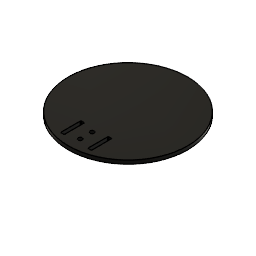
Mirror Mount v1 (Autodesk Fusion 360 design; units mm, degrees)
part number: 2026-03-18-09-30-07-770
Autodesk Fusion 360 part; units mm, degrees
note: some values were not read from the file. Set by a fixed rule: which sketch regions a step uses.
sketch "Sketch1" plane through (0, 0, 0) normal (0, 1, 0) x (1, 0, 0)
  circle A0 centre (0, 0) radius 27.5
  circle A1 centre (0, 0) radius 25
  circle A2 centre (0, 0) radius 50
  circle A3 centre (0, 0) radius 24
  line L0 (0, 0) -> (24, 0)
  dimension "d1" = 55
  dimension "d2" = 50
  dimension "d3" = 100
  dimension "d6" = 48
  constraint coincident A0.centre A1.centre
  constraint concentric A0 A3
  constraint coincident A3 L0.end
  constraint horizontal L0
  measures "d1" diameter of A0
  measures "d2" diameter of A1
  measures "d3" diameter of A2
  measures "d6" diameter of A3
extrude "Extrude2" add sketch "Sketch1" along normal blind 3 contours A0 | A1 | A2 | A3 picked at (26.564283, -1.366221) picked at (24.484237, -2.434357) picked at (42.211463, -3.850259) picked at (3.644582, 2.6578) makes body 1
sketch "Sketch2" plane through (0, 0, 0) normal (0, 0, 1) x (1, 0, 0)
  line L0 (0, 0) -> (0, -14.937)
  line L1 (24, 0) -> (0, -14.937)
  line L2 (0, 0) -> (24, 0)
  line L3 (-1, 1) -> (-1, -16.737233)
  line L4 (27.499271, 1) -> (-1, -16.737233)
  line L5 (-1, 1) -> (27.499271, 1)
  line L6 (0, -14.937) -> (0, -16.114858)
  line L7 (24, 0) -> (25.892523, 0)
  dimension "d9" = 14.937
  dimension "d21" = -1
  constraint coincident L0.start L2.start
  constraint vertical L0
  constraint perpendicular L0 L2
  constraint parallel L0 L6
  constraint perpendicular L6 L7
  measures "d9" distance of L0.start L0.end
revolve "Revolve1" add sketch "Sketch2" angle 360 about axis through (0, 0, 0) along (0, -1, 0) contours L0 L1 L2 picked at (8, -4.979) bodies 1
sketch "Sketch3" plane through (0, 3, 0) normal (0, 1, 0) x (-1, 0, 0)
  circle A0 centre (0, 0) radius 50
  line L0 (0, 0) -> (0, -25)
  circle A1 centre (0, -25) radius 20
  line L1 (0, 0) -> (0, 35)
  line L2 (0, 35) -> (0, 30)
  line L3 (0, 35) -> (0, 40)
  circle A2 centre (0, 40) radius 1.65
  circle A3 centre (0, 30) radius 1.65
  dimension "d11" = 25
  dimension "d12" = 40
  dimension "d13" = 35
  dimension "d14" = 5
  dimension "d15" = 5
  dimension "d16" = 3.3
  dimension "d17" = 3.3
  constraint coincident A0.centre L0.start
  constraint vertical L0
  constraint coincident L0.end A1.centre
  constraint parallel L0 L1
  constraint parallel L1 L2
  constraint parallel L1 L3
  constraint coincident L3.end A2.centre
  constraint coincident L2.end A3.centre
  measures "d11" distance of A0.centre L0.end
  measures "d12" diameter of A1
  measures "d13" distance of A0.centre L1.end
  measures "d14" distance of L1.end L2.end
  measures "d15" distance of L1.end L3.end
  measures "d16" diameter of A2
  measures "d17" diameter of A3
extrude "Extrude3" cut sketch "Sketch3" against normal blind 4 contours L1 L2 A3 | L1 L2 A3 | A2 picked at (-0.906321, 29.382081) picked at (1.072123, 29.766774) picked at (-0.523888, 40.740498) bodies 1
revolve "Revolve2" add sketch "Sketch2" angle 360 about axis through (0, 1.75, 0) along (0, 1, 0) separate body contours L1 L4 L6 L7 picked at (16.630841, -5.371619) makes body 2
extrude "Extrude4" add 1 faces at (-0.023343, 3, -23.789631) along direction (0, 1, 0) blind 5 on bodies 1 bodies 1
sketch "Sketch4" plane through (0, 0, 0) normal (0, -1, 0) x (1, 0, 0)
  circle A0 centre (0, 0) radius 24
  circle A1 centre (0, 0) radius 50
  circle A2 centre (0, 0) radius 24
  circle A3 centre (0, 0) radius 50
  circle A4 centre (0, 30) radius 1.65
  circle A5 centre (0, 40) radius 1.65
  line L0 (0, 30) -> (0, 40)
  line L1 (11.43, 35) -> (-11.43, 35)
  line L2 (11.43, 35) -> (11.43, 43.5)
  line L3 (11.43, 43.5) -> (12.93, 43.5)
  line L4 (12.93, 43.5) -> (9.93, 43.5)
  line L5 (9.93, 43.5) -> (9.93, 26.5)
  line L6 (9.93, 26.5) -> (12.93, 26.5)
  line L7 (12.93, 26.5) -> (12.93, 43.5)
  line L8 (-9.93, 43.5) -> (-9.93, 26.5)
  line L9 (-12.93, 26.5) -> (-12.93, 43.5)
  line L10 (-9.93, 26.5) -> (-12.93, 26.5)
  line L11 (-12.93, 43.5) -> (-9.93, 43.5)
  line L12 (12.93, 43.5) -> (9.93, 43.5)
  line L13 (9.93, 43.5) -> (9.93, 26.5)
  line L14 (9.93, 26.5) -> (12.93, 26.5)
  line L15 (12.93, 26.5) -> (12.93, 43.5)
  point P0 (0, 35)
  dimension "d25" = 48
  dimension "d30" = 22.86
  dimension "d31" = 8.5
  dimension "d32" = 1.5
  dimension "d33" = 3
  dimension "d34" = 17
  constraint coincident A0.centre A1.centre
  constraint concentric A2 A3
  constraint coincident A4.centre L0.start
  constraint coincident A5.centre L0.end
  constraint midpoint L1 P0
  constraint coincident L0 P0
  constraint perpendicular L0 L1
  constraint perpendicular L1 L2
  constraint perpendicular L2 L3
  constraint horizontal L4
  constraint vertical L5
  constraint horizontal L6
  constraint vertical L7
  constraint symmetric L0 L3.end L9.end
  constraint symmetric L0 L4.end L8.start
  constraint symmetric L0 L5.end L8.end
  constraint symmetric L0 L6.end L9.start
  constraint horizontal L12
  constraint vertical L13
  constraint horizontal L14
  constraint vertical L15
  measures "d25" diameter of A2
  measures "d30" distance of L1.start L1.end
  measures "d31" distance of L1.start L2.end
  measures "d32" distance of L2.end L3.end
  measures "d33" distance of L3.end L4.end
  measures "d34" distance of L3.end L6.end
extrude "Extrude5" cut sketch "Sketch4" against normal blind 5 contours A1 A3 | A4 | A5 | L1 L2 L3 L4 L5 L6 L7 L12 L13 L14 L15 | L1 L2 L4 L5 L12 L13 | L8 L9 L10 L11 picked at (-22.391946, 25.610928) picked at (0.414083, 30.418311) picked at (-0.523888, 40.740498) picked at (11.43, 29.333333) picked at (10.43, 37.833333) picked at (-11.93, 35) bodies 1
extrude "Extrude6" cut 1 faces at (-9.530328, 5, 33.144779) along direction (0, -1, 0) blind 20 on bodies 1 bodies 2
extrude "Extrude7" cut sketch "Sketch4" against normal blind 26 contours L1 L2 L3 L4 L5 L6 L7 L12 L13 L14 L15 | L1 L2 L4 L5 L12 L13 | L8 L9 L10 L11 picked at (11.43, 29.333333) picked at (10.43, 37.833333) picked at (-11.93, 35) bodies 1
fillet "Fillet1" radius 0.5 8 edges at (-12.93, 6.5, 26.5) (-9.93, 6.5, 26.5) (-12.93, 6.5, 43.5) (-9.93, 6.5, 43.5) (9.93, 6.5, 26.5) (9.93, 6.5, 43.5) (12.93, 6.5, 43.5) (12.93, 6.5, 26.5) on bodies 1
